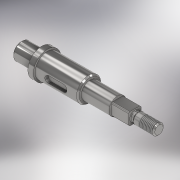
# Autodesk Inventor part: 零件1
Saved by Autodesk Inventor 2020 (Build 240168000, 168)
## iProperties
Created: 2021-04-14
Part Number: 零件1
Material: 钢，高强度，低合金
Document SubType Name: Modeling
Designer: Luorily
Density: 7.85 g/cm^3
Appearance: 钢 - 抛光
Author: Luorily
Autodesk Inventor part; units mm, degrees
ref_plane "YZ Plane" through (0, 0, 0) normal (1, 0, 0) x (0, 1, 0)
ref_plane "XZ Plane" through (0, 0, 0) normal (0, 1, 0) x (-1, 0, 0)
sketch "草图1" plane through (0, 0, 0) normal (0, 0, 1) x (1, 0, 0)
  line L0 (0, 0) -> (220, 0)
  line L1 (0, 0) -> (0, 12.5)
  line L2 (0, 12.5) -> (30, 12.5)
  line L3 (30, 12.5) -> (30, 20)
  line L4 (30, 20) -> (38, 20)
  line L5 (38, 20) -> (38, 17.5)
  line L6 (38, 17.5) -> (100, 17.5)
  line L7 (100, 17.5) -> (100, 12.5)
  line L8 (100, 12.5) -> (140, 12.5)
  line L9 (140, 12.5) -> (140, 0)
  dimension "d0" = 220
  dimension "d1" = 12.5
  dimension "d2" = 30
  dimension "d3" = 7.5
  dimension "d4" = 8
  dimension "d5" = 2.5
  dimension "d6" = 62
  dimension "d7" = 5
  dimension "d8" = 40
  constraints: 20 end point, 6 perpendicular, 3 point on line, 1 horizontal, 1 vertical
  measures "d0" distance of L0.start L0.end
  measures "d1" distance of L0.start L1.end
  measures "d2" distance of L1.end L2.end
  measures "d3" distance of L2.end L3.end
  measures "d4" distance of L3.end L4.end
  measures "d5" distance of L4.end L5.end
  measures "d6" distance of L5.end L6.end
  measures "d7" distance of L6.end L7.end
  measures "d8" distance of L7.end L8.end
revolve "旋转1" add sketch "草图1" angle 360 about axis through (0, 0, 0) along (1, 0, 0)
sketch "草图2" plane through (140, 0, 0) normal (1, 0, 0) x (0, 0, -1)
  circle A0 centre (0, 0) radius 12.5 projected
  line L0 (0, 9) -> (-9, 9)
  line L1 (-9, 9) -> (-9, -9)
  line L2 (-9, -9) -> (9, -9)
  line L3 (9, -9) -> (9, 9)
  line L4 (9, 9) -> (0, 9)
  arc A1 (9, 7.1589) -> (7.1589, 9) centre (0, 0) ccw
  arc A2 (7.1589, -9) -> (9, -7.1589) centre (0, 0) ccw
  arc A3 (-7.1589, 9) -> (-9, 7.1589) centre (0, 0) ccw
  arc A4 (-9, -7.1589) -> (-7.1589, -9) centre (0, 0) ccw
  point P0 (8.6747, 9)
  point P1 (-8.6747, 9)
  point P2 (-9, 8.6747)
  point P3 (-9, -8.6747)
  point P4 (-8.6747, -9)
  point P5 (8.6747, -9)
  point P6 (9, -8.6747)
  point P7 (9, 8.6747)
  dimension "d13" = 9
  dimension "d14" = 18
  dimension "d15" = 18
  dimension "d16" = 18
  constraints: 10 end point, 9 point on line, 8 point on circle, 4 centre point, 2 perpendicular, 1 coincident
  measures "d13" distance of L0.start L0.end
  measures "d14" distance of L0.end L1.end
  measures "d15" distance of L1.end L2.end
  measures "d16" distance of L2.end L3.end
extrude "拉伸2" add sketch "草图2" along normal blind 25 contours L3 A2 L2 A4 L1 A3 L0 L4 A1
sketch "草图3" plane through (165, 0, 0) normal (1, 0, 0) x (0, 0, -1)
  arc A0 (-9, -7.1589) -> (-7.1589, -9) centre (0, 0) ccw projected
  circle A1 centre (0, 0) radius 6.5
  dimension "d22" = 13
  constraints: 2 coincident, 1 centre point
  measures "d22" diameter of A1
extrude "拉伸3" add sketch "草图3" along normal blind 6
sketch "草图4" plane through (171, 0, 0) normal (1, 0, 0) x (0, 0, -1)
  circle A0 centre (0, 0) radius 6.5 projected
  circle A1 centre (0, 0) radius 8
  dimension "d25" = 16
  constraints: 1 centre point, 1 coincident
  measures "d25" diameter of A1
extrude "拉伸4" add sketch "草图4" along normal blind 29 contours A0 | A1
thread "螺纹1" size "M16x2" class "6g" standard "ANSI Metric M Profile" length 22 offset 7
chamfer "倒角1" distance 2 angle 45 3 edges at (200, 0, 8) (100, -17.5, 0) (0, -12.5, 0)
fillet "圆角1" radius 1 1 edges at (165, 0, 6.5)
ref_plane "工作平面1" through (0, 0, 17.5) normal (0, 0, 1) x (1, 0, 0)
sketch "草图5" plane through (0, 0, 17.5) normal (0, 0, 1) x (1, 0, 0)
  line L0 (100, -12.5) -> (100, 12.5) projected
  line L1 (79, 5) -> (57, 5)
  line L2 (57, -5) -> (79, -5)
  arc A0 (57, 5) -> (57, -5) centre (57, 0) ccw
  arc A1 (79, -5) -> (79, 5) centre (79, 0) ccw
  point P0 (0, 0)
  constraints: 4 end point, 4 point on circle, 2 centre point
extrude "拉伸5" cut sketch "草图5" against normal blind 5
sketch "草图6" plane through (171, 0, 0) normal (-1, 0, 0) x (0, 0, 1)
  circle A0 centre (0, 0) radius 8 projected
  circle A1 centre (0, 0) radius 6.5 projected
extrude "拉伸6" add sketch "草图6" along normal blind 1.5
chamfer "倒角2" distance 1.5 angle 45 1 edges at (169.5, 0, -8)
fillet "圆角2" radius 1 2 edges at (169.5, 0, -6.5001) (169.5, 0, 6.5)
